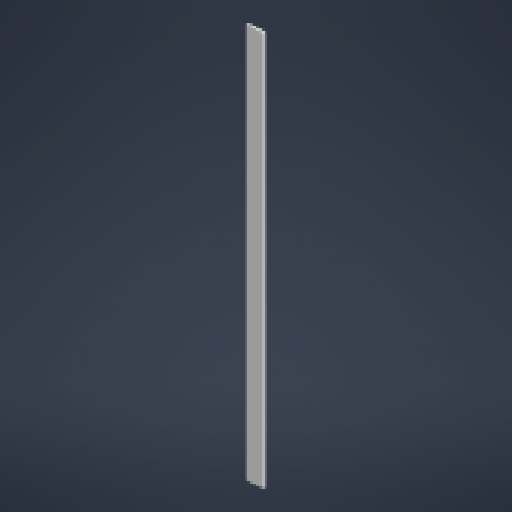
# Autodesk Inventor part: SuperstructureStrut_1
Saved by Autodesk Inventor 2024 (Build 280153000, 153)
## iProperties
Created: 2025-03-18
Part Number: SuperstructureStrut_1
Material: Steel, Alloy
Document SubType Name: Sheet Metal
Designer: Tommy Rohmann
Density: 7.73 g/cm^3
Appearance: Semi-Polished
Sheet Metal Rule: Default
Author: Tommy Rohmann
Autodesk Inventor part; units mm, degrees
ref_plane "YZ Plane" through (0, 0, 0) normal (1, 0, 0) x (0, 1, 0)
ref_plane "XZ Plane" through (0, 0, 0) normal (0, 1, 0) x (-1, 0, 0)
ref_plane "XY Plane" through (0, 0, 0) normal (0, 0, 1) x (1, 0, 0)
sketch "SuperstructureStrut" plane through (0, 0, 0) normal (0, 0, 1) x (1, 0, 0)
  line L0 (-903.0105, 0) -> (-925.2355, 0)
  line L1 (-925.2355, 0) -> (-925.2355, 544.83)
  line L2 (-925.2355, 544.83) -> (-903.0105, 544.83)
  line L3 (-903.0105, 544.83) -> (-903.0105, 0)
  point P0 (-914.123, 272.415)
  dimension "d622" = 22.225
  dimension "d623" = 544.83
  measures "d622" distance of L0.start L0.end
  measures "d623" distance of L0.end L1.end
derived "LAYOUT.ipt"
sketch "Sketch1" plane through (0, 0, 0) normal (0, 0, 1) x (1, 0, 0)
  line L0 (-903.0105, 0) -> (-925.2355, 0)
  line L1 (-925.2355, 0) -> (-925.2355, 544.83)
  line L2 (-925.2355, 544.83) -> (-903.0105, 544.83)
  line L3 (-903.0105, 544.83) -> (-903.0105, 0)
extrude "Plate1" add sketch "Sketch1" along normal blind 3.175
equation "\"d1\" = Thickness"
equation "\"BendRadius\" = Thickness"
equation "\"BendReliefWidth\" = Thickness"
equation "\"BendReliefDepth\" = 0.5 * Thickness"
equation "\"CornerReliefSize\" = 4 * Thickness"
equation "\"MinimumRemnant\" = 2 * Thickness"
equation "\"TransitionRadius\" = BendRadius"
equation "\"JacobiRadiusSize\" = BendRadius"
equation "\"GapSize\" = Thickness"
equation "\"Thickness\" = 3.175"
body "Solid1"
